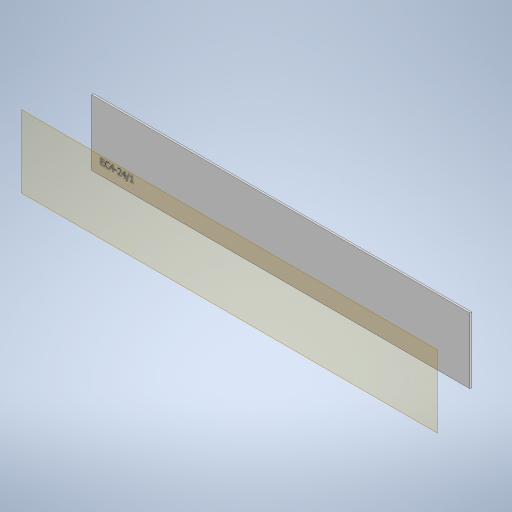
# Autodesk Inventor part: Fechamento
Saved by Autodesk Inventor 2024.2 (Build 282272000, 272)
## iProperties
Created: 2024-05-06
Part Number: Fechamento
Material: Generic
Document SubType Name: Modeling
Designer: 082220019
Density: 1 g/cm^3
Appearance: Default
Author: 082220019
Autodesk Inventor part; units mm, degrees
ref_plane "YZ Plane" through (0, 0, 0) normal (1, 0, 0) x (0, 1, 0)
ref_plane "XZ Plane" through (0, 0, 0) normal (0, 1, 0) x (-1, 0, 0)
ref_plane "XY Plane" through (0, 0, 0) normal (0, 0, 1) x (1, 0, 0)
sketch "Sketch1" plane through (0, 0, 0) normal (0, 0, 1) x (1, 0, 0)
  line L0 (0, 0) -> (1905, 0)
  line L1 (1905, 0) -> (1905, 330.2)
  line L2 (1905, 330.2) -> (0, 330.2)
  line L3 (0, 330.2) -> (0, 0)
  dimension "d0" = 330.2
  dimension "d1" = 1905
  constraints: 8 end point, 2 parallel, 1 horizontal, 1 perpendicular
  measures "d0" distance of L0.end L1.end
  measures "d1" distance of L1.end L2.end
extrude "Extrusion1" add sketch "Sketch1" along normal blind 9.0322
ref_plane "Work Plane1" through (0, 0, 267.7947) normal (0, 0, 1) x (1, 0, 0)
sketch "Sketch2" plane through (0, 0, 267.7947) normal (0, 0, 1) x (1, 0, 0)
  line L0 (42.5276, 79.6263) -> (256.0708, 79.6263) construction
  line L1 (256.0708, 79.6263) -> (256.0708, 19.9066) construction
  line L2 (256.0708, 19.9066) -> (42.5276, 19.9066) construction
  line L3 (42.5276, 19.9066) -> (42.5276, 79.6263) construction
  line L4 (45.6152, 47.7877) -> (45.6152, 78.2677)
  line L5 (45.6152, 78.2677) -> (64.6837, 78.2677)
  line L6 (64.6837, 78.2677) -> (64.6837, 74.6615)
  line L7 (64.6837, 74.6615) -> (49.666, 74.6615)
  line L8 (49.666, 74.6615) -> (49.666, 66.3129)
  line L9 (49.666, 66.3129) -> (63.671, 66.3129)
  line L10 (63.671, 66.3129) -> (63.671, 62.7066)
  line L11 (63.671, 62.7066) -> (49.666, 62.7066)
  line L12 (49.666, 62.7066) -> (49.666, 51.394)
  line L13 (49.666, 51.394) -> (64.6837, 51.394)
  line L14 (64.6837, 51.394) -> (64.6837, 47.7877)
  line L15 (64.6837, 47.7877) -> (45.6152, 47.7877)
  spline S0 degree 2 poles (81.0352, 47.2443) (78.0712, 47.2443) (73.057, 49.245) (71.2292, 51.2458) knots 0 0 0 1 2 2 2
  spline S1 degree 2 poles (71.2292, 51.2458) (69.4014, 53.2218) (67.4007, 59.1498) (67.4007, 63.003) knots 0 0 0 1 2 2 2
  spline S2 degree 2 poles (67.4007, 63.003) (67.4007, 66.8316) (69.352, 72.5126) (71.2045, 74.6121) knots 0 0 0 1 2 2 2
  spline S3 degree 2 poles (71.2045, 74.6121) (73.0323, 76.6622) (78.0218, 78.8111) (81.1093, 78.8111) knots 0 0 0 1 2 2 2
  spline S4 degree 2 poles (81.1093, 78.8111) (82.6407, 78.8111) (85.333, 78.3665) (86.4692, 78.0207) knots 0 0 0 1 2 2 2
  spline S5 degree 2 poles (86.4692, 78.0207) (87.4572, 77.6996) (89.5073, 76.7857) (90.52, 76.2423) knots 0 0 0 1 2 2 2
  line L16 (90.52, 76.2423) -> (90.52, 71.3517)
  line L17 (90.52, 71.3517) -> (90.1989, 71.3517)
  spline S6 degree 2 poles (90.1989, 71.3517) (89.6555, 71.8457) (87.9759, 73.2289) (86.7656, 73.8958) knots 0 0 0 1 2 2 2
  spline S7 degree 2 poles (86.7656, 73.8958) (85.6047, 74.538) (82.863, 75.3531) (81.0846, 75.3531) knots 0 0 0 1 2 2 2
  spline S8 degree 2 poles (81.0846, 75.3531) (79.1333, 75.3531) (75.6505, 73.7476) (74.3414, 72.2162) knots 0 0 0 1 2 2 2
  spline S9 degree 2 poles (74.3414, 72.2162) (73.057, 70.6601) (71.6244, 65.9424) (71.6244, 63.003) knots 0 0 0 1 2 2 2
  spline S10 degree 2 poles (71.6244, 63.003) (71.6244, 59.8661) (73.1311, 55.346) (74.4402, 53.7899) knots 0 0 0 1 2 2 2
  spline S11 degree 2 poles (74.4402, 53.7899) (75.7246, 52.2832) (79.158, 50.7518) (81.0846, 50.7518) knots 0 0 0 1 2 2 2
  spline S12 degree 2 poles (81.0846, 50.7518) (82.8383, 50.7518) (85.827, 51.6163) (86.9879, 52.2585) knots 0 0 0 1 2 2 2
  spline S13 degree 2 poles (86.9879, 52.2585) (88.0994, 52.9007) (89.7543, 54.2345) (90.2236, 54.7038) knots 0 0 0 1 2 2 2
  line L18 (90.2236, 54.7038) -> (90.52, 54.7038)
  line L19 (90.52, 54.7038) -> (90.52, 49.8626)
  spline S14 degree 2 poles (90.52, 49.8626) (89.5073, 49.3933) (87.7289, 48.5287) (86.4692, 48.1335) knots 0 0 0 1 2 2 2
  spline S15 degree 2 poles (86.4692, 48.1335) (85.1354, 47.6889) (82.863, 47.2443) (81.0352, 47.2443) knots 0 0 0 1 2 2 2
  line L20 (113.0466, 58.2606) -> (109.4157, 58.2606)
  line L21 (109.4157, 58.2606) -> (109.4157, 47.7877)
  line L22 (109.4157, 47.7877) -> (105.4883, 47.7877)
  line L23 (105.4883, 47.7877) -> (105.4883, 58.2606)
  line L24 (105.4883, 58.2606) -> (92.0268, 58.2606)
  line L25 (92.0268, 58.2606) -> (92.0268, 62.5584)
  line L26 (92.0268, 62.5584) -> (105.6612, 78.2677)
  line L27 (105.6612, 78.2677) -> (109.4157, 78.2677)
  line L28 (109.4157, 78.2677) -> (109.4157, 61.5457)
  line L29 (109.4157, 61.5457) -> (113.0466, 61.5457)
  line L30 (113.0466, 61.5457) -> (113.0466, 58.2606)
  line L31 (105.4883, 61.5457) -> (105.4883, 73.4512)
  line L32 (105.4883, 73.4512) -> (95.2378, 61.5457)
  line L33 (95.2378, 61.5457) -> (105.4883, 61.5457)
  line L34 (127.4715, 59.2733) -> (115.9365, 59.2733)
  line L35 (115.9365, 59.2733) -> (115.9365, 62.9783)
  line L36 (115.9365, 62.9783) -> (127.4715, 62.9783)
  line L37 (127.4715, 62.9783) -> (127.4715, 59.2733)
  line L38 (150.3191, 47.7877) -> (131.5223, 47.7877)
  line L39 (131.5223, 47.7877) -> (131.5223, 52.1103)
  spline S16 degree 2 poles (131.5223, 52.1103) (133.5477, 54.0122) (137.154, 57.5443) (138.883, 59.4462) knots 0 0 0 1 2 2 2
  spline S17 degree 2 poles (138.883, 59.4462) (142.3657, 63.2747) (144.9098, 67.869) (144.9098, 70.3143) knots 0 0 0 1 2 2 2
  spline S18 degree 2 poles (144.9098, 70.3143) (144.9098, 71.5987) (144.1194, 73.5253) (143.4031, 74.1428) knots 0 0 0 1 2 2 2
  spline S19 degree 2 poles (143.4031, 74.1428) (142.6868, 74.7603) (140.8096, 75.3778) (139.6734, 75.3778) knots 0 0 0 1 2 2 2
  spline S20 degree 2 poles (139.6734, 75.3778) (138.5866, 75.3778) (136.3635, 74.8344) (135.3508, 74.4145) knots 0 0 0 1 2 2 2
  spline S21 degree 2 poles (135.3508, 74.4145) (134.4863, 74.0687) (132.8808, 73.0807) (132.3868, 72.7349) knots 0 0 0 1 2 2 2
  line L40 (132.3868, 72.7349) -> (132.1645, 72.7349)
  line L41 (132.1645, 72.7349) -> (132.1645, 77.0821)
  spline S22 degree 2 poles (132.1645, 77.0821) (133.4242, 77.6996) (137.9444, 78.9099) (139.9698, 78.9099) knots 0 0 0 1 2 2 2
  spline S23 degree 2 poles (139.9698, 78.9099) (144.2429, 78.9099) (149.0594, 74.3898) (149.0594, 70.5366) knots 0 0 0 1 2 2 2
  spline S24 degree 2 poles (149.0594, 70.5366) (149.0594, 68.7335) (148.2196, 65.7201) (147.4786, 64.4356) knots 0 0 0 1 2 2 2
  spline S25 degree 2 poles (147.4786, 64.4356) (146.7376, 63.1018) (144.5887, 60.4836) (143.4031, 59.2239) knots 0 0 0 1 2 2 2
  spline S26 degree 2 poles (143.4031, 59.2239) (141.4765, 57.1244) (136.7588, 52.629) (135.3508, 51.3199) knots 0 0 0 1 2 2 2
  line L42 (135.3508, 51.3199) -> (150.3191, 51.3199)
  line L43 (150.3191, 51.3199) -> (150.3191, 47.7877)
  line L44 (174.0066, 58.2606) -> (170.3757, 58.2606)
  line L45 (170.3757, 58.2606) -> (170.3757, 47.7877)
  line L46 (170.3757, 47.7877) -> (166.4483, 47.7877)
  line L47 (166.4483, 47.7877) -> (166.4483, 58.2606)
  line L48 (166.4483, 58.2606) -> (152.9868, 58.2606)
  line L49 (152.9868, 58.2606) -> (152.9868, 62.5584)
  line L50 (152.9868, 62.5584) -> (166.6212, 78.2677)
  line L51 (166.6212, 78.2677) -> (170.3757, 78.2677)
  line L52 (170.3757, 78.2677) -> (170.3757, 61.5457)
  line L53 (170.3757, 61.5457) -> (174.0066, 61.5457)
  line L54 (174.0066, 61.5457) -> (174.0066, 58.2606)
  line L55 (166.4483, 61.5457) -> (166.4483, 73.4512)
  line L56 (166.4483, 73.4512) -> (156.1978, 61.5457)
  line L57 (156.1978, 61.5457) -> (166.4483, 61.5457)
  line L58 (189.9382, 79.6263) -> (178.008, 41.1681)
  line L59 (178.008, 41.1681) -> (174.55, 41.1681)
  line L60 (174.55, 41.1681) -> (186.4308, 79.6263)
  line L61 (186.4308, 79.6263) -> (189.9382, 79.6263)
  line L62 (210.5628, 47.7877) -> (195.6933, 47.7877)
  line L63 (195.6933, 47.7877) -> (195.6933, 50.9)
  line L64 (195.6933, 50.9) -> (201.2262, 50.9)
  line L65 (201.2262, 50.9) -> (201.2262, 71.327)
  line L66 (201.2262, 71.327) -> (195.6933, 71.327)
  line L67 (195.6933, 71.327) -> (195.6933, 74.1181)
  spline S27 degree 2 poles (195.6933, 74.1181) (198.8303, 74.1181) (201.7943, 75.8965) (201.9919, 78.3665) knots 0 0 0 1 2 2 2
  line L68 (201.9919, 78.3665) -> (205.1535, 78.3665)
  line L69 (205.1535, 78.3665) -> (205.1535, 50.9)
  line L70 (205.1535, 50.9) -> (210.5628, 50.9)
  line L71 (210.5628, 50.9) -> (210.5628, 47.7877)
  point P0 (0, 0)
  constraints: 2 other
emboss "Emboss1" sketch "Sketch2" operation cut depth 7.62 direction (0, 0, -1)
body "Solid1"
